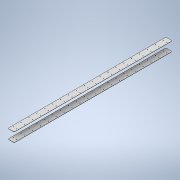
# Autodesk Inventor part: side_panels_for_beam_v2
Saved by Autodesk Inventor 2022 (Build 260153000, 153)
## iProperties
Created: 2022-04-07
Part Number: side_panels_for_beam_v2
Material: Generic
Document SubType Name: Sheet Metal
Designer: marcu
Density: 1 g/cm^3
Sheet Metal Rule: Default_mm
Appearance: Default
Author: marcu
Autodesk Inventor part; units mm, degrees
ref_plane "YZ Plane" through (0, 0, 0) normal (1, 0, 0) x (0, 1, 0)
ref_plane "XZ Plane" through (0, 0, 0) normal (0, 1, 0) x (-1, 0, 0)
ref_plane "XY Plane" through (0, 0, 0) normal (0, 0, 1) x (1, 0, 0)
sketch "Sketch1" plane through (0, 0, 0) normal (0, 1, 0) x (-1, 0, 0)
  line L0 (0, 0) -> (40, 0)
  line L1 (40, 0) -> (40, -1000)
  line L2 (40, -1000) -> (0, -1000)
  line L3 (0, -1000) -> (0, 0)
  line L4 (40, -1000) -> (20, -1000)
  line L5 (20, -1000) -> (20, 0)
  line L6 (31, -1000) -> (31, 0)
  circle A0 centre (31, -975) radius 1.675
  dimension "d0" = 1000
  dimension "d1" = 40
  dimension "d10" = 20
  dimension "d11" = 11
  dimension "d12" = 3.35
  dimension "d13" = 25
  measures "d0" distance of L0.end L1.end
  measures "d1" distance of L1.end L2.end
  measures "d10" distance between parallel lines of L3 L5
  measures "d11" distance between parallel lines of L5 L6
  measures "d12" diameter of A0
  measures "d13" distance of L6.start A0.centre
extrude "Plate1" add sketch "Sketch1" along normal blind 1.5
fillet "Corner Round1" radius 6 4 edges at (-40, 0.75, 0) (0, 0.75, 0) (0, 0.75, -1000) (-40, 0.75, -1000)
move or copy body "Move Body2" bodies to move or copy 1 copy no translate (0, -30, 0)
sketch "Sketch3" plane through (-34, -30, -1000) normal (0, -1, 0) x (1, 0, 0)
  circle A0 centre (25, 25) radius 1.675
  line L0 (34, 6) -> (34, 994) projected
  line L1 (0, 0) -> (28, 0) projected
  point P0 (34, 1000)
  dimension "d19" = 9
  dimension "d20" = 25
  dimension "d21" = 3.35
  constraints: 1 centre point
  measures "d19" distance from line of A0.centre L0
  measures "d20" distance from line of L1 A0.centre
  measures "d21" diameter of A0
extrude "Extrusion2" cut sketch "Sketch3" against normal blind 10
pattern_linear "Rectangular Pattern1" count 20 spacing 50 along (0, 0, 1) count 2 spacing 22 along (-1, 0, 0) of "Extrusion2"
mirror "Mirror2" about plane through (0, 0, 0) normal (0, 1, 0)
equation "\"d2\" = Thickness"
equation "\"BendRadius\" = Thickness"
equation "\"BendReliefWidth\" = Thickness"
equation "\"BendReliefDepth\" = 0.5 * Thickness"
equation "\"CornerReliefSize\" = 4 * Thickness"
equation "\"MinimumRemnant\" = 2 * Thickness"
equation "\"TransitionRadius\" = BendRadius"
equation "\"JacobiRadiusSize\" = BendRadius"
equation "\"GapSize\" = Thickness"
equation "\"Thickness\" = 1.5"
body "Solid1"
